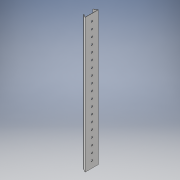
# Autodesk Inventor part: Thing1
Saved by Autodesk Inventor 2018 (Build 220112000, 112)
## iProperties
Created: 2017-11-20
Part Number: Thing1
Material: Generic
Document SubType Name: Modeling
Designer: ash-pc
Density: 1 g/cm^3
Appearance: Default
Author: ash-pc
Autodesk Inventor part; units mm, degrees
ref_plane "YZ Plane" through (0, 0, 0) normal (1, 0, 0) x (0, 1, 0)
ref_plane "XZ Plane" through (0, 0, 0) normal (0, 1, 0) x (-1, 0, 0)
ref_plane "XY Plane" through (0, 0, 0) normal (0, 0, 1) x (1, 0, 0)
sketch "Sketch1" plane through (0, 0, 0) normal (0, 1, 0) x (-1, 0, 0)
  line L0 (0, 0) -> (0, 12.7)
  line L1 (0, 12.7) -> (3.2996, 10.795)
  line L2 (0, 0) -> (3.2996, 1.905)
  line L3 (0, 0) -> (3.81, 0) construction
  line L4 (3.1726, 10.575) -> (0.254, 12.2601)
  line L5 (0.254, 12.2601) -> (0.254, 0.4399)
  line L6 (0.254, 0.4399) -> (3.1726, 2.125)
  line L7 (3.1726, 10.575) -> (3.2996, 10.795)
  line L8 (3.1726, 2.125) -> (3.2996, 1.905)
  dimension "d0" = 12.7
  dimension "d1" = 3.81
  dimension "d2" = 60
  dimension "d3" = 30
  dimension "d4" = 0.254
  constraints: 18 end point, 1 equal length, 1 horizontal, 1 vertical, 2 other
  measures "d0" distance of L0.start L0.end
  measures "d1" distance of L0.end L1.end
  measures "d2" angle of L0 L1
  measures "d3" angle of L3 L2
  measures "d4" distance between parallel lines of L0 L5
extrude "Extrusion1" add sketch "Sketch1" along normal blind 127
sketch "Sketch2" plane through (-0.254, 0, 0.4399) normal (-1, 0, 0) x (0, 0, 1)
  line L0 (5.2751, 5.715) -> (6.5451, 5.715)
  line L1 (6.5451, 5.715) -> (6.5451, 6.985)
  line L2 (6.5451, 6.985) -> (5.2751, 6.985)
  line L3 (5.2751, 6.985) -> (5.2751, 5.715)
  line L4 (5.2751, 5.715) -> (6.5451, 6.985) construction
  line L5 (6.5451, 5.715) -> (5.2751, 6.985) construction
  line L6 (6.5451, 12.065) -> (6.5451, 13.335)
  line L7 (6.5451, 13.335) -> (5.2751, 13.335)
  line L8 (5.2751, 13.335) -> (5.2751, 12.065)
  line L9 (5.2751, 12.065) -> (6.5451, 12.065)
  line L10 (6.5451, 18.415) -> (6.5451, 19.685)
  line L11 (6.5451, 19.685) -> (5.2751, 19.685)
  line L12 (5.2751, 19.685) -> (5.2751, 18.415)
  line L13 (5.2751, 18.415) -> (6.5451, 18.415)
  line L14 (6.5451, 24.765) -> (6.5451, 26.035)
  line L15 (6.5451, 26.035) -> (5.2751, 26.035)
  line L16 (5.2751, 26.035) -> (5.2751, 24.765)
  line L17 (5.2751, 24.765) -> (6.5451, 24.765)
  line L18 (6.5451, 31.115) -> (6.5451, 32.385)
  line L19 (6.5451, 32.385) -> (5.2751, 32.385)
  line L20 (5.2751, 32.385) -> (5.2751, 31.115)
  line L21 (5.2751, 31.115) -> (6.5451, 31.115)
  line L22 (6.5451, 37.465) -> (6.5451, 38.735)
  line L23 (6.5451, 38.735) -> (5.2751, 38.735)
  line L24 (5.2751, 38.735) -> (5.2751, 37.465)
  line L25 (5.2751, 37.465) -> (6.5451, 37.465)
  line L26 (6.5451, 43.815) -> (6.5451, 45.085)
  line L27 (6.5451, 45.085) -> (5.2751, 45.085)
  line L28 (5.2751, 45.085) -> (5.2751, 43.815)
  line L29 (5.2751, 43.815) -> (6.5451, 43.815)
  line L30 (6.5451, 50.165) -> (6.5451, 51.435)
  line L31 (6.5451, 51.435) -> (5.2751, 51.435)
  line L32 (5.2751, 51.435) -> (5.2751, 50.165)
  line L33 (5.2751, 50.165) -> (6.5451, 50.165)
  line L34 (6.5451, 56.515) -> (6.5451, 57.785)
  line L35 (6.5451, 57.785) -> (5.2751, 57.785)
  line L36 (5.2751, 57.785) -> (5.2751, 56.515)
  line L37 (5.2751, 56.515) -> (6.5451, 56.515)
  line L38 (6.5451, 62.865) -> (6.5451, 64.135)
  line L39 (6.5451, 64.135) -> (5.2751, 64.135)
  line L40 (5.2751, 64.135) -> (5.2751, 62.865)
  line L41 (5.2751, 62.865) -> (6.5451, 62.865)
  line L42 (6.5451, 69.215) -> (6.5451, 70.485)
  line L43 (6.5451, 70.485) -> (5.2751, 70.485)
  line L44 (5.2751, 70.485) -> (5.2751, 69.215)
  line L45 (5.2751, 69.215) -> (6.5451, 69.215)
  line L46 (6.5451, 75.565) -> (6.5451, 76.835)
  line L47 (6.5451, 76.835) -> (5.2751, 76.835)
  line L48 (5.2751, 76.835) -> (5.2751, 75.565)
  line L49 (5.2751, 75.565) -> (6.5451, 75.565)
  line L50 (6.5451, 81.915) -> (6.5451, 83.185)
  line L51 (6.5451, 83.185) -> (5.2751, 83.185)
  line L52 (5.2751, 83.185) -> (5.2751, 81.915)
  line L53 (5.2751, 81.915) -> (6.5451, 81.915)
  line L54 (6.5451, 88.265) -> (6.5451, 89.535)
  line L55 (6.5451, 89.535) -> (5.2751, 89.535)
  line L56 (5.2751, 89.535) -> (5.2751, 88.265)
  line L57 (5.2751, 88.265) -> (6.5451, 88.265)
  line L58 (6.5451, 94.615) -> (6.5451, 95.885)
  line L59 (6.5451, 95.885) -> (5.2751, 95.885)
  line L60 (5.2751, 95.885) -> (5.2751, 94.615)
  line L61 (5.2751, 94.615) -> (6.5451, 94.615)
  line L62 (6.5451, 100.965) -> (6.5451, 102.235)
  line L63 (6.5451, 102.235) -> (5.2751, 102.235)
  line L64 (5.2751, 102.235) -> (5.2751, 100.965)
  line L65 (5.2751, 100.965) -> (6.5451, 100.965)
  line L66 (6.5451, 107.315) -> (6.5451, 108.585)
  line L67 (6.5451, 108.585) -> (5.2751, 108.585)
  line L68 (5.2751, 108.585) -> (5.2751, 107.315)
  line L69 (5.2751, 107.315) -> (6.5451, 107.315)
  line L70 (6.5451, 113.665) -> (6.5451, 114.935)
  line L71 (6.5451, 114.935) -> (5.2751, 114.935)
  line L72 (5.2751, 114.935) -> (5.2751, 113.665)
  line L73 (5.2751, 113.665) -> (6.5451, 113.665)
  line L74 (6.5451, 120.015) -> (6.5451, 121.285)
  line L75 (6.5451, 121.285) -> (5.2751, 121.285)
  line L76 (5.2751, 121.285) -> (5.2751, 120.015)
  line L77 (5.2751, 120.015) -> (6.5451, 120.015)
  point P0 (-0.4399, 0)
  point P1 (5.9101, 6.35)
  dimension "d7" = 1.27
  dimension "d8" = 1.27
  dimension "d14" = 6.35
  constraints: 156 end point, 2 midpoint, 2 parallel, 1 collinear, 1 horizontal, 1 perpendicular, 1 vertical, 143 other
  measures "d7" distance of L2.end L1.end
  measures "d8" distance of L1.end L0.end
  measures "d14" distance of L0.end L6.start
extrude "Extrusion2" cut sketch "Sketch2" against normal blind 0.254
body "Solid1"
